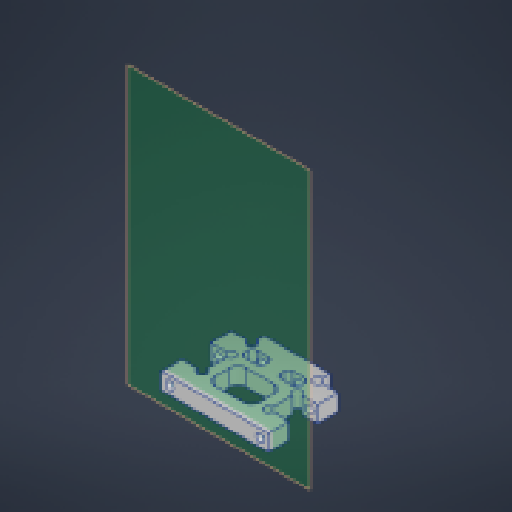
# Autodesk Inventor part: Roll_Fixation_Frameto64
Saved by Autodesk Inventor 2024 (Build 280153000, 153)
## iProperties
Created: 2024-01-23
Part Number: Roll_Fixation_Frameto64
Material: 알루미늄 6061
Document SubType Name: Modeling
Designer: ASUS
Density: 2.7 g/cm^3
Appearance: 알루미늄 - 평지
Author: ASUS
Autodesk Inventor part; units mm, degrees
ref_plane "작업 평면1" through (0, 37, 16) normal (0, 0, -1) x (-1, 0, 0)
sketch "스케치1" plane through (0, 37, 16) normal (0, 0, -1) x (-1, 0, 0)
  arc A0 (20.1, 4.5766) -> (19.5808, 6.2636) centre (17.1, 4.5766) ccw projected
  line L0 (19.5808, 6.2636) -> (15.5953, 12.1246) projected
  arc A1 (15.5953, 12.1246) -> (13.9414, 13) centre (13.9414, 11) ccw projected
  line L1 (13, 13) -> (13.9414, 13) projected
  arc A2 (14.5, 11.5) -> (13, 13) centre (13, 11.5) ccw projected
  line L2 (14.5, -41.5) -> (14.5, 11.5) projected
  arc A3 (13.5, -42.5) -> (14.5, -41.5) centre (13.5, -41.5) ccw projected
  line L3 (-13.5, -42.5) -> (13.5, -42.5) projected
  arc A4 (-14.5, -41.5) -> (-13.5, -42.5) centre (-13.5, -41.5) ccw projected
  line L4 (-14.5, 11.5) -> (-14.5, -41.5) projected
  arc A5 (-13, 13) -> (-14.5, 11.5) centre (-13, 11.5) ccw projected
  line L5 (-13.9414, 13) -> (-13, 13) projected
  arc A6 (-13.9414, 13) -> (-15.5953, 12.1246) centre (-13.9414, 11) ccw projected
  line L6 (-15.5953, 12.1246) -> (-19.5808, 6.2636) projected
  arc A7 (-19.5808, 6.2636) -> (-20.1, 4.5766) centre (-17.1, 4.5766) ccw projected
  line L7 (-20.1, 4.5766) -> (-20.1, -39.6766) projected
  arc A8 (-20.1, -39.6766) -> (-19.5808, -41.3636) centre (-17.1, -39.6766) ccw projected
  line L8 (-19.5808, -41.3636) -> (-15.8929, -46.7869) projected
  arc A9 (-15.8929, -46.7869) -> (-13.4121, -48.1) centre (-13.4121, -45.1) ccw projected
  line L9 (-13.4121, -48.1) -> (13.4121, -48.1) projected
  arc A10 (13.4121, -48.1) -> (15.8929, -46.7869) centre (13.4121, -45.1) ccw projected
  line L10 (15.8929, -46.7869) -> (19.5808, -41.3636) projected
  arc A11 (19.5808, -41.3636) -> (20.1, -39.6766) centre (17.1, -39.6766) ccw projected
  line L11 (20.1, -39.6766) -> (20.1, 4.5766) projected
  circle A12 centre (-17.3, 4) radius 1.35 projected
  circle A13 centre (-17.3, -18) radius 1.35 projected
  circle A14 centre (-11, -45.3) radius 1.35 projected
  circle A15 centre (17.3, 4) radius 1.35 projected
  circle A16 centre (17.3, -18) radius 1.35 projected
  circle A17 centre (11, -45.3) radius 1.35 projected
  circle A18 centre (-17.3, -40) radius 1.35 projected
  circle A19 centre (17.3, -40) radius 1.35 projected
  line L12 (-7.1991, -36.7384) -> (-5.2861, -28.9475) projected
  arc A20 (-2.675, -27.5395) -> (-5.2861, -28.9475) centre (-3.3438, -29.4244) ccw projected
  arc A21 (-2.675, -27.5395) -> (2.675, -27.5395) centre (0, -20) ccw projected
  arc A22 (5.2861, -28.9475) -> (2.675, -27.5395) centre (3.3438, -29.4244) ccw projected
  line L13 (5.2861, -28.9475) -> (7.1991, -36.7384) projected
  arc A23 (5.8409, -39.1281) -> (7.1991, -36.7384) centre (5.2568, -37.2153) ccw projected
  arc A24 (-5.8409, -39.1281) -> (5.8409, -39.1281) centre (0, -20) ccw projected
  arc A25 (-7.1991, -36.7384) -> (-5.8409, -39.1281) centre (-5.2568, -37.2153) ccw projected
  circle A26 centre (11, -45.3) radius 1.35 projected
  circle A27 centre (-11, -45.3) radius 1.35 projected
  arc A28 (-4, -43.3) -> (-8, -43.3) centre (-6, -43.3) ccw projected
  line L14 (-4, -43.3) -> (4, -43.3) projected
  arc A29 (8, -43.3) -> (4, -43.3) centre (6, -43.3) ccw projected
  line L15 (8, -43.3) -> (8, -47.3) projected
  arc A30 (4, -47.3) -> (8, -47.3) centre (6, -47.3) ccw projected
  line L16 (4, -47.3) -> (-4, -47.3) projected
  arc A31 (-8, -47.3) -> (-4, -47.3) centre (-6, -47.3) ccw projected
  line L17 (-8, -47.3) -> (-8, -43.3) projected
  line L18 (16.3659, -53.1031) -> (7.7692, -18.0923) projected
  arc A32 (7.7692, -18.0923) -> (-7.7692, -18.0923) centre (0, -20) ccw projected
  line L19 (-7.7692, -18.0923) -> (-16.3659, -53.1031) projected
  arc A33 (-16.3659, -53.1031) -> (-16.539, -54.5339) centre (-10.539, -54.5339) ccw projected
  line L20 (-16.539, -54.5339) -> (-16.539, -62.05) projected
  arc A34 (-16.539, -62.05) -> (-10.539, -68.05) centre (-10.539, -62.05) ccw projected
  line L21 (-10.539, -68.05) -> (10.539, -68.05) projected
  arc A35 (10.539, -68.05) -> (16.539, -62.05) centre (10.539, -62.05) ccw projected
  line L22 (16.539, -62.05) -> (16.539, -54.5339) projected
  arc A36 (16.539, -54.5339) -> (16.3659, -53.1031) centre (10.539, -54.5339) ccw projected
  circle A37 centre (10.539, -60) radius 1.35 projected
  circle A38 centre (-10.461, -60) radius 1.35 projected
  circle A39 centre (0, -20) radius 4 projected
  line L23 (-3.961, -62) -> (4.039, -62) projected
  arc A40 (-7.461, -62) -> (-3.961, -62) centre (-5.711, -62) ccw projected
  line L24 (-7.461, -58) -> (-7.461, -62) projected
  arc A41 (-3.961, -58) -> (-7.461, -58) centre (-5.711, -58) ccw projected
  line L25 (4.039, -58) -> (-3.961, -58) projected
  arc A42 (7.539, -58) -> (4.039, -58) centre (5.789, -58) ccw projected
  line L26 (7.539, -62) -> (7.539, -58) projected
  arc A43 (4.039, -62) -> (7.539, -62) centre (5.789, -62) ccw projected
  line L27 (13, -43.3) -> (9, -43.3)
  line L28 (9, -43.3) -> (9, -47.3)
  line L29 (9, -47.3) -> (13, -47.3)
  line L30 (13, -47.3) -> (13, -43.3)
  line L31 (13, -43.3) -> (9, -47.3) construction
  line L32 (9, -43.3) -> (13, -47.3) construction
  line L33 (-9, -43.3) -> (-13, -43.3)
  line L34 (-13, -43.3) -> (-13, -47.3)
  line L35 (-13, -47.3) -> (-9, -47.3)
  line L36 (-9, -47.3) -> (-9, -43.3)
  line L37 (-9, -43.3) -> (-13, -47.3) construction
  line L38 (-13, -43.3) -> (-9, -47.3) construction
  line L39 (13, -47.3) -> (-13, -47.3)
  line L40 (-13, -47.3) -> (-13, -43.3)
  line L41 (-13, -43.3) -> (13, -43.3)
  line L42 (13, -43.3) -> (13, -47.3)
  line L43 (4, -47.3) -> (-4, -47.3)
  line L44 (-4, -47.3) -> (-4, -43.3)
  line L45 (-4, -43.3) -> (4, -43.3)
  line L46 (4, -43.3) -> (4, -47.3)
  point P0 (0, -37)
  point P1 (4, -47.3)
  point P2 (4, -43.3)
  point P3 (-4, -43.3)
  dimension "d0" = 4
  dimension "d1" = 4
  dimension "d2" = 4
  dimension "d3" = 4
  constraints: 40 end point, 8 parallel, 4 horizontal, 4 midpoint, 4 perpendicular
  measures "d0" distance of L29.end L28.end
  measures "d1" distance of L28.end L27.end
  measures "d2" distance of L35.end L34.end
  measures "d3" distance of L34.end L33.end
ref_plane "작업 평면2" through (-16.539, -31.05, 0) normal (0, 0, 1) x (1, 0, 0)
extrude "돌출1" add sketch "스케치1" along normal up to surface (16 mm away) contours L39 L46 L41 L15 | L15 L41 L28 L39 | L16 L44 L14 L46 | L28 L27 L30 L29 | L39 L17 L41 L44 | L39 L36 L41 L17 | L35 L34 L33 L36
sketch "스케치2" plane through (13, -6.3, 0) normal (0, 0, -1) x (-1, 0, 0)
  line L0 (5.8009, 6.5616) -> (7.7139, 14.3525) projected
  arc A0 (10.325, 15.7605) -> (7.7139, 14.3525) centre (9.6562, 13.8756) ccw projected
  arc A1 (10.325, 15.7605) -> (15.675, 15.7605) centre (13, 23.3) ccw projected
  arc A2 (18.2861, 14.3525) -> (15.675, 15.7605) centre (16.3438, 13.8756) ccw projected
  line L1 (18.2861, 14.3525) -> (20.1991, 6.5616) projected
  arc A3 (18.8409, 4.1719) -> (20.1991, 6.5616) centre (18.2568, 6.0847) ccw projected
  arc A4 (7.1591, 4.1719) -> (18.8409, 4.1719) centre (13, 23.3) ccw projected
  arc A5 (5.8009, 6.5616) -> (7.1591, 4.1719) centre (7.7432, 6.0847) ccw projected
  circle A6 centre (24, -2) radius 1.35 projected
  circle A7 centre (2, -2) radius 1.35 projected
  arc A8 (9, 0) -> (5, 0) centre (7, 0) ccw projected
  line L2 (9, 0) -> (17, 0) projected
  arc A9 (21, 0) -> (17, 0) centre (19, 0) ccw projected
  line L3 (21, 0) -> (21, -4) projected
  arc A10 (17, -4) -> (21, -4) centre (19, -4) ccw projected
  line L4 (17, -4) -> (9, -4) projected
  arc A11 (5, -4) -> (9, -4) centre (7, -4) ccw projected
  line L5 (5, -4) -> (5, 0) projected
  line L6 (29.3659, -9.8031) -> (20.7692, 25.2077) projected
  arc A12 (20.7692, 25.2077) -> (5.2308, 25.2077) centre (13, 23.3) ccw projected
  line L7 (5.2308, 25.2077) -> (-3.3659, -9.8031) projected
  arc A13 (-3.3659, -9.8031) -> (-3.539, -11.2339) centre (2.461, -11.2339) ccw projected
  line L8 (-3.539, -11.2339) -> (-3.539, -18.75) projected
  arc A14 (-3.539, -18.75) -> (2.461, -24.75) centre (2.461, -18.75) ccw projected
  line L9 (2.461, -24.75) -> (23.539, -24.75) projected
  arc A15 (23.539, -24.75) -> (29.539, -18.75) centre (23.539, -18.75) ccw projected
  line L10 (29.539, -18.75) -> (29.539, -11.2339) projected
  arc A16 (29.539, -11.2339) -> (29.3659, -9.8031) centre (23.539, -11.2339) ccw projected
  circle A17 centre (23.539, -16.7) radius 1.35 projected
  circle A18 centre (2.539, -16.7) radius 1.35 projected
  circle A19 centre (13, 23.3) radius 4 projected
  line L11 (9.039, -18.7) -> (17.039, -18.7) projected
  arc A20 (5.539, -18.7) -> (9.039, -18.7) centre (7.289, -18.7) ccw projected
  line L12 (5.539, -14.7) -> (5.539, -18.7) projected
  arc A21 (9.039, -14.7) -> (5.539, -14.7) centre (7.289, -14.7) ccw projected
  line L13 (17.039, -14.7) -> (9.039, -14.7) projected
  arc A22 (20.539, -14.7) -> (17.039, -14.7) centre (18.789, -14.7) ccw projected
  line L14 (20.539, -18.7) -> (20.539, -14.7) projected
  arc A23 (17.039, -18.7) -> (20.539, -18.7) centre (18.789, -18.7) ccw projected
  line L15 (21, -4) -> (5, -4)
  line L16 (5, -4) -> (5, 0)
  line L17 (5, 0) -> (21, 0)
  line L18 (21, 0) -> (21, -4)
  point P0 (13, 6.3)
  point P1 (21, 0)
  point P2 (17, 0)
  point P3 (9, 0)
  point P4 (5, -4)
  point P5 (9, -4)
  point P6 (17, -4)
  constraints: 8 end point, 2 parallel, 1 horizontal, 1 perpendicular
ref_plane "작업 평면3" through (-16.539, -31.05, -2) normal (0, 0, -1) x (0, 1, 0)
extrude "돌출2" add sketch "스케치2" along normal up to surface (2 mm away) contours L2 L17 L3 L15 L4 L5
sketch "스케치3" plane through (-13, -10.3, 16) normal (0, -1, 0) x (1, 0, 0)
  line L0 (26, -16) -> (21, -16) projected
  line L1 (26, 0) -> (26, -16) projected
  line L2 (26, 0) -> (0, 0) projected
  line L3 (0, 0) -> (0, -16) projected
  line L4 (5, -16) -> (0, -16) projected
  line L5 (5, -16) -> (5, -18) projected
  line L6 (5, -18) -> (21, -18) projected
  line L7 (21, -16) -> (21, -18) projected
  circle A0 centre (5, -16) radius 1.1
  line L8 (21, -16) -> (21, -18) projected
  circle A1 centre (21, -16) radius 1.1
  point P0 (13, -16)
  dimension "d8" = 2.2
  dimension "d9" = 2.2
  constraints: 2 centre point, 2 coincident
  measures "d8" diameter of A0
  measures "d9" diameter of A1
extrude "돌출3" cut sketch "스케치3" against normal through all contours A1 L7 L0 | L0 L7 A1 | A0 L5 L4 | L4 L5 A0
sketch "스케치4" plane through (8, -6.3, -2) normal (0, 0, -1) x (-1, 0, 0)
  line L0 (16, 0) -> (16, -4) projected
  line L1 (0, 0) -> (16, 0) projected
  line L2 (0, -4) -> (0, 0) projected
  line L3 (16, -4) -> (0, -4) projected
  line L4 (16, -4) -> (16, 0) projected
  line L5 (16, -2) -> (0, -2)
  circle A0 centre (8, -2) radius 1
  circle A1 centre (8, -2) radius 2.5
  line L6 (17.1, -4) -> (14.9, -4) projected
  line L7 (1.1, -4) -> (-1.1, -4) projected
  line L8 (14.9, -4) -> (1.1, -4)
  line L9 (1.1, -4) -> (1.1, 0)
  line L10 (1.1, 0) -> (14.9, 0)
  line L11 (14.9, 0) -> (14.9, -4)
  line L12 (16, -4) -> (0, -4) projected
  circle A2 centre (-13.2666, 1.4722) radius 1
  circle A3 centre (-13.2666, 1.4722) radius 2.5
  line L13 (-13.2666, 1.4722) -> (-15.7666, 1.4722)
  line L14 (-13.2666, 1.4722) -> (-10.7666, 1.4722)
  circle A4 centre (14.9, -2) radius 0.5
  circle A5 centre (1.1, -2) radius 0.5
  circle A6 centre (12.4, -2) radius 1
  circle A7 centre (12.4, -2) radius 2.5
  line L15 (12.4, -2) -> (9.9, -2)
  line L16 (12.4, -2) -> (14.9, -2)
  circle A8 centre (3.6, -2) radius 1
  circle A9 centre (3.6, -2) radius 2.5
  line L17 (3.6, -2) -> (1.1, -2)
  line L18 (3.6, -2) -> (6.1, -2)
  point P0 (8, 6.3)
  dimension "d12" = 2
  dimension "d13" = 5
  dimension "d14" = 2
  dimension "d15" = 5
  dimension "d16" = 1
  dimension "d17" = 1
  dimension "d18" = 2
  dimension "d19" = 5
  dimension "d20" = 2
  dimension "d21" = 5
  constraints: 22 end point, 10 centre point, 6 horizontal, 6 point on circle, 5 midpoint, 4 coincident, 2 parallel, 1 collinear, 1 perpendicular
  measures "d12" diameter of A0
  measures "d13" diameter of A1
  measures "d14" diameter of A2
  measures "d15" diameter of A3
  measures "d16" diameter of A4
  measures "d17" diameter of A5
  measures "d18" diameter of A6
  measures "d19" diameter of A7
  measures "d20" diameter of A8
  measures "d21" diameter of A9
extrude "돌출4" cut sketch "스케치4" against normal blind 10 contours A6 L5 | L5 A6 | A8 L5 | L5 A8
sketch "스케치5" plane through (-13, -10.3, 0) normal (0, 0, -1) x (-1, 0, 0)
  circle A0 centre (-2, 2) radius 1.35 projected
  circle A1 centre (-24, 2) radius 1.35 projected
  line L0 (-20.1991, 10.5616) -> (-18.2861, 18.3525) projected
  arc A2 (-15.675, 19.7605) -> (-18.2861, 18.3525) centre (-16.3438, 17.8756) ccw projected
  arc A3 (-15.675, 19.7605) -> (-10.325, 19.7605) centre (-13, 27.3) ccw projected
  arc A4 (-7.7139, 18.3525) -> (-10.325, 19.7605) centre (-9.6562, 17.8756) ccw projected
  line L1 (-7.7139, 18.3525) -> (-5.8009, 10.5616) projected
  arc A5 (-7.1591, 8.1719) -> (-5.8009, 10.5616) centre (-7.7432, 10.0847) ccw projected
  arc A6 (-18.8409, 8.1719) -> (-7.1591, 8.1719) centre (-13, 27.3) ccw projected
  arc A7 (-20.1991, 10.5616) -> (-18.8409, 8.1719) centre (-18.2568, 10.0847) ccw projected
  circle A8 centre (-2, 2) radius 1.35 projected
  circle A9 centre (-24, 2) radius 1.35 projected
  arc A10 (-17, 4) -> (-21, 4) centre (-19, 4) ccw projected
  line L2 (-17, 4) -> (-9, 4) projected
  arc A11 (-5, 4) -> (-9, 4) centre (-7, 4) ccw projected
  line L3 (-5, 4) -> (-5, 0) projected
  arc A12 (-9, 0) -> (-5, 0) centre (-7, 0) ccw projected
  line L4 (-9, 0) -> (-17, 0) projected
  arc A13 (-21, 0) -> (-17, 0) centre (-19, 0) ccw projected
  line L5 (-21, 0) -> (-21, 4) projected
  line L6 (3.3659, -5.8031) -> (-5.2308, 29.2077) projected
  arc A14 (-5.2308, 29.2077) -> (-20.7692, 29.2077) centre (-13, 27.3) ccw projected
  line L7 (-20.7692, 29.2077) -> (-29.3659, -5.8031) projected
  arc A15 (-29.3659, -5.8031) -> (-29.539, -7.2339) centre (-23.539, -7.2339) ccw projected
  line L8 (-29.539, -7.2339) -> (-29.539, -14.75) projected
  arc A16 (-29.539, -14.75) -> (-23.539, -20.75) centre (-23.539, -14.75) ccw projected
  line L9 (-23.539, -20.75) -> (-2.461, -20.75) projected
  arc A17 (-2.461, -20.75) -> (3.539, -14.75) centre (-2.461, -14.75) ccw projected
  line L10 (3.539, -14.75) -> (3.539, -7.2339) projected
  arc A18 (3.539, -7.2339) -> (3.3659, -5.8031) centre (-2.461, -7.2339) ccw projected
  circle A19 centre (-2.461, -12.7) radius 1.35 projected
  circle A20 centre (-23.461, -12.7) radius 1.35 projected
  circle A21 centre (-13, 27.3) radius 4 projected
  line L11 (-16.961, -14.7) -> (-8.961, -14.7) projected
  arc A22 (-20.461, -14.7) -> (-16.961, -14.7) centre (-18.711, -14.7) ccw projected
  line L12 (-20.461, -10.7) -> (-20.461, -14.7) projected
  arc A23 (-16.961, -10.7) -> (-20.461, -10.7) centre (-18.711, -10.7) ccw projected
  line L13 (-8.961, -10.7) -> (-16.961, -10.7) projected
  arc A24 (-5.461, -10.7) -> (-8.961, -10.7) centre (-7.211, -10.7) ccw projected
  line L14 (-5.461, -14.7) -> (-5.461, -10.7) projected
  arc A25 (-8.961, -14.7) -> (-5.461, -14.7) centre (-7.211, -14.7) ccw projected
  circle A26 centre (-24, 2) radius 1
  circle A27 centre (-2, 2) radius 1
  point P0 (-13, 10.3)
  dimension "d24" = 2
  dimension "d25" = 2
  constraints: 2 centre point, 2 coincident
  measures "d24" diameter of A26
  measures "d25" diameter of A27
ref_plane "작업 평면4" through (-20.1, -11.1, 16) normal (0, 0, -1) x (0, 1, 0)
extrude "돌출5" add sketch "스케치5" against normal up to surface (16 mm away) contours A0 | A1
sketch "스케치6" plane through (-13, -10.3, 16) normal (0, -1, 0) x (1, 0, 0)
  arc A0 (22.1, -16) -> (21, -17.1) centre (21, -16) ccw projected
  line L0 (26, -16) -> (22.1, -16) projected
  line L1 (26, 0) -> (26, -16) projected
  line L2 (26, 0) -> (0, 0) projected
  line L3 (0, 0) -> (0, -16) projected
  line L4 (3.9, -16) -> (0, -16) projected
  arc A1 (5, -17.1) -> (3.9, -16) centre (5, -16) ccw projected
  line L5 (5, -17.1) -> (5, -18) projected
  line L6 (5, -18) -> (21, -18) projected
  line L7 (21, -17.1) -> (21, -18) projected
  line L8 (0, 0) -> (26, 0)
  line L9 (26, 0) -> (26, -16)
  line L10 (26, -16) -> (0, -16)
  line L11 (0, -16) -> (0, 0)
  line L12 (3.5, -12.5) -> (22.5, -12.5)
  line L13 (22.5, -12.5) -> (22.5, -3.5)
  line L14 (22.5, -3.5) -> (3.5, -3.5)
  line L15 (3.5, -3.5) -> (3.5, -12.5)
  point P0 (13, -16)
  dimension "d28" = 3.5
  constraints: 16 end point, 4 parallel, 2 perpendicular, 1 horizontal, 3 other
  measures "d28" distance between parallel lines of L10 L12
extrude "돌출6" cut sketch "스케치6" against normal through all contours L15 L14 L13 L12
sketch "스케치7" plane through (-13, -10.3, 16) normal (0, -1, 0) x (1, 0, 0)
  line L0 (3.5, -3.5) -> (22.5, -3.5) projected
  line L1 (22.5, -3.5) -> (22.5, -12.5) projected
  line L2 (22.5, -12.5) -> (3.5, -12.5) projected
  line L3 (3.5, -12.5) -> (3.5, -3.5) projected
  arc A0 (22.1, -16) -> (21, -17.1) centre (21, -16) ccw projected
  line L4 (26, -16) -> (22.1, -16) projected
  line L5 (26, 0) -> (26, -16) projected
  line L6 (26, 0) -> (0, 0) projected
  line L7 (0, 0) -> (0, -16) projected
  line L8 (3.9, -16) -> (0, -16) projected
  arc A1 (5, -17.1) -> (3.9, -16) centre (5, -16) ccw projected
  line L9 (5, -17.1) -> (5, -18) projected
  line L10 (5, -18) -> (21, -18) projected
  line L11 (21, -17.1) -> (21, -18) projected
  line L12 (3.5, -12.5) -> (13, -3.5)
  line L13 (22.5, -12.5) -> (13, -3.5)
  line L14 (4.1877, -13.226) -> (13, -4.8775)
  line L15 (13, -4.8775) -> (21.8123, -13.226)
  line L16 (2.8123, -11.774) -> (13, -2.1225)
  line L17 (13, -2.1225) -> (23.1877, -11.774)
  point P0 (13, -16)
  point P1 (11.546, -3.5)
  point P2 (3.5, -11.1225)
  point P3 (4.954, -12.5)
  point P4 (21.046, -12.5)
  point P5 (22.5, -11.1225)
  point P6 (14.454, -3.5)
  dimension "d31" = 1
  dimension "d32" = 1
  constraints: 12 end point, 1 midpoint, 2 other
  measures "d31" distance between parallel lines of L12 L14
  measures "d32" distance between parallel lines of L12 L16
extrude "돌출7" add sketch "스케치7" against normal up to surface (4 mm away) contours L0 L12 L3 L16 | L13 L2 L15 L14 L12 | L0 L17 L1 L13
fillet "모깎기1" radius 1 9 edges at (-9.5, -8.3, 12.5) (-9.5, -8.3, 4.8775) (-1.454, -8.3, 12.5) (0, -8.3, 11.1225) (1.454, -8.3, 12.5) (9.5, -8.3, 12.5) (9.5, -8.3, 4.8775) (8.046, -8.3, 3.5) (-8.046, -8.3, 3.5)
sketch "스케치8" plane through (0, 37, 16) normal (0, 0, 1) x (1, 0, 0)
  circle A0 centre (11, -45.3) radius 1 projected
  circle A1 centre (-11, -45.3) radius 1 projected
  line L0 (-13, -43.3) -> (13, -43.3) projected
  line L1 (-13, -47.3) -> (-13, -43.3) projected
  line L2 (13, -47.3) -> (-13, -47.3) projected
  line L3 (13, -43.3) -> (13, -47.3) projected
  point P0 (0, -37)
extrude "돌출8" add sketch "스케치8" along normal blind 1
sketch "스케치9" plane through (8, -6.3, -2) normal (0, 0, -1) x (-1, 0, 0)
  circle A0 centre (3.6, -2) radius 1 projected
  circle A1 centre (12.4, -2) radius 1 projected
  line L0 (16, 0) -> (16, -4) projected
  line L1 (0, 0) -> (16, 0) projected
  line L2 (0, -4) -> (0, 0) projected
  line L3 (16, -4) -> (0, -4) projected
  point P0 (8, 6.3)
ref_plane "작업 평면5" through (-21.6156, -28.6331, -3) normal (0, 0, -1) x (0, 1, 0)
extrude "돌출9" add sketch "스케치9" along normal up to surface (1 mm away)
sketch "스케치10" plane through (9.1, -10.3, 0) normal (0, -1, 0) x (1, 0, 0)
  line L0 (-5.1364, 12.5) -> (-0.6, 12.5) projected
  arc A0 (0.4, 11.5) -> (-0.6, 12.5) centre (-0.6, 11.5) ccw projected
  line L1 (0.4, 11.5) -> (0.4, 7.2024) projected
  arc A1 (-1.2877, 6.4764) -> (0.4, 7.2024) centre (-0.6, 7.2024) ccw projected
  line L2 (-1.2877, 6.4764) -> (-5.8241, 10.774) projected
  arc A2 (-5.1364, 12.5) -> (-5.8241, 10.774) centre (-5.1364, 11.5) ccw projected
  line L3 (-12.3759, 10.774) -> (-16.9123, 6.4764) projected
  arc A3 (-18.6, 7.2024) -> (-16.9123, 6.4764) centre (-17.6, 7.2024) ccw projected
  line L4 (-18.6, 7.2024) -> (-18.6, 11.5) projected
  arc A4 (-17.6, 12.5) -> (-18.6, 11.5) centre (-17.6, 11.5) ccw projected
  line L5 (-17.6, 12.5) -> (-13.0636, 12.5) projected
  arc A5 (-12.3759, 10.774) -> (-13.0636, 12.5) centre (-13.0636, 11.5) ccw projected
  line L6 (-15.3241, 5.226) -> (-9.7877, 10.471) projected
  arc A6 (-8.4123, 10.471) -> (-9.7877, 10.471) centre (-9.1, 9.745) ccw projected
  line L7 (-8.4123, 10.471) -> (-2.8759, 5.226) projected
  arc A7 (-3.5636, 3.5) -> (-2.8759, 5.226) centre (-3.5636, 4.5) ccw projected
  line L8 (-3.5636, 3.5) -> (-14.6364, 3.5) projected
  arc A8 (-15.3241, 5.226) -> (-14.6364, 3.5) centre (-14.6364, 4.5) ccw projected
  arc A9 (0, 0) -> (-1.1, -1.1) centre (-1.1, 0) ccw projected
  line L9 (3.9, 0) -> (0, 0) projected
  line L10 (3.9, 17) -> (3.9, 0) projected
  line L11 (-22.1, 17) -> (3.9, 17) projected
  line L12 (-22.1, 17) -> (-22.1, 0) projected
  line L13 (-18.2, 0) -> (-22.1, 0) projected
  arc A10 (-17.1, -1.1) -> (-18.2, 0) centre (-17.1, 0) ccw projected
  line L14 (-17.1, -1.1) -> (-17.1, -3) projected
  line L15 (-17.1, -3) -> (-1.1, -3) projected
  line L16 (-1.1, -1.1) -> (-1.1, -3) projected
  point P0 (-9.1, 0)
extrude "돌출10" add sketch "스케치10" against normal up to surface (4 mm away) contours L0 A0 L1 A1 L2 A2 | L3 A3 L4 A4 L5 A5 | L6 A6 L7 A7 L8 A8
sketch "스케치11" plane through (9.1, -10.3, 0) normal (0, -1, 0) x (1, 0, 0)
  line L0 (-19.1, 0) -> (-21.1, 0) projected
  line L1 (2.9, 0) -> (0.9, 0) projected
  arc A0 (0, 0) -> (-1.1, -1.1) centre (-1.1, 0) ccw projected
  line L2 (3.9, 0) -> (0, 0) projected
  line L3 (3.9, 17) -> (3.9, 0) projected
  line L4 (-22.1, 17) -> (3.9, 17) projected
  line L5 (-22.1, 17) -> (-22.1, 0) projected
  line L6 (-18.2, 0) -> (-22.1, 0) projected
  arc A1 (-17.1, -1.1) -> (-18.2, 0) centre (-17.1, 0) ccw projected
  line L7 (-17.1, -1.1) -> (-17.1, -3) projected
  line L8 (-17.1, -3) -> (-1.1, -3) projected
  line L9 (-1.1, -1.1) -> (-1.1, -3) projected
  line L10 (-22.1, 17) -> (-22.1, 0) projected
  line L11 (-22.1, 17) -> (-22.1, 0)
  line L12 (-22.1, 0) -> (-20.1, 0)
  line L13 (-20.1, 0) -> (-20.1, 17)
  line L14 (-20.1, 17) -> (-22.1, 17)
  line L15 (3.9, 17) -> (3.9, 0)
  line L16 (3.9, 0) -> (1.9, 0)
  line L17 (1.9, 0) -> (1.9, 17)
  line L18 (1.9, 17) -> (3.9, 17)
  line L19 (-22.1, 0) -> (-20.1, 0)
  line L20 (-20.1, 0) -> (-20.1, 5)
  line L21 (-20.1, 5) -> (-22.1, 5)
  line L22 (-22.1, 5) -> (-22.1, 0)
  line L23 (-22.1, 17) -> (3.9, 17) projected
  line L24 (-20.1, 17) -> (-22.1, 17)
  line L25 (-22.1, 17) -> (-22.1, 12)
  line L26 (-22.1, 12) -> (-20.1, 12)
  line L27 (-20.1, 12) -> (-20.1, 17)
  line L28 (1.9, 17) -> (3.9, 17)
  line L29 (3.9, 17) -> (3.9, 12)
  line L30 (3.9, 12) -> (1.9, 12)
  line L31 (1.9, 12) -> (1.9, 17)
  line L32 (1.9, 0) -> (3.9, 0)
  line L33 (3.9, 0) -> (3.9, 5)
  line L34 (3.9, 5) -> (1.9, 5)
  line L35 (1.9, 5) -> (1.9, 0)
  line L36 (-18.1, 10.5) -> (-22.1, 10.5)
  line L37 (-22.1, 10.5) -> (-22.1, 13.5)
  line L38 (-22.1, 13.5) -> (-18.1, 13.5)
  line L39 (-18.1, 13.5) -> (-18.1, 10.5)
  line L40 (-18.1, 10.5) -> (-22.1, 13.5) construction
  line L41 (-22.1, 10.5) -> (-18.1, 13.5) construction
  line L42 (-22.1, 5) -> (-20.1, 5)
  line L43 (-18.1, 3.5) -> (-22.1, 3.5)
  line L44 (-22.1, 3.5) -> (-22.1, 6.5)
  line L45 (-22.1, 6.5) -> (-18.1, 6.5)
  line L46 (-18.1, 6.5) -> (-18.1, 3.5)
  line L47 (-18.1, 3.5) -> (-22.1, 6.5) construction
  line L48 (-22.1, 3.5) -> (-18.1, 6.5) construction
  line L49 (-0.1, 5) -> (1.9, 5)
  line L50 (3.9, 3.5) -> (-0.1, 3.5)
  line L51 (-0.1, 3.5) -> (-0.1, 6.5)
  line L52 (-0.1, 6.5) -> (3.9, 6.5)
  line L53 (3.9, 6.5) -> (3.9, 3.5)
  line L54 (3.9, 3.5) -> (-0.1, 6.5) construction
  line L55 (-0.1, 3.5) -> (3.9, 6.5) construction
  line L56 (-0.1, 12) -> (1.9, 12)
  line L57 (3.9, 10.5) -> (-0.1, 10.5)
  line L58 (-0.1, 10.5) -> (-0.1, 13.5)
  line L59 (-0.1, 13.5) -> (3.9, 13.5)
  line L60 (3.9, 13.5) -> (3.9, 10.5)
  line L61 (3.9, 10.5) -> (-0.1, 13.5) construction
  line L62 (-0.1, 10.5) -> (3.9, 13.5) construction
  line L63 (-22.1, 13.5) -> (-22.1, 10.5)
  line L64 (-22.1, 10.5) -> (-17.1, 10.5)
  line L65 (-17.1, 10.5) -> (-17.1, 13.5)
  line L66 (-17.1, 13.5) -> (-22.1, 13.5)
  line L67 (-22.1, 6.5) -> (-22.1, 3.5)
  line L68 (-22.1, 3.5) -> (3.9, 3.5)
  line L69 (3.9, 3.5) -> (3.9, 6.5)
  line L70 (3.9, 6.5) -> (-22.1, 6.5)
  line L71 (3.9, 3.5) -> (3.9, 6.5)
  line L72 (3.9, 6.5) -> (-1.1, 6.5)
  line L73 (-1.1, 6.5) -> (-1.1, 3.5)
  line L74 (-1.1, 3.5) -> (3.9, 3.5)
  line L75 (3.9, 13.5) -> (3.9, 10.5)
  line L76 (3.9, 10.5) -> (-1.1, 10.5)
  line L77 (-1.1, 10.5) -> (-1.1, 13.5)
  line L78 (-1.1, 13.5) -> (3.9, 13.5)
  line L79 (-17.1, 13.5) -> (-1.1, 13.5)
  line L80 (-1.1, 13.5) -> (-1.1, 3.5)
  line L81 (-1.1, 3.5) -> (-17.1, 3.5)
  line L82 (-17.1, 3.5) -> (-17.1, 13.5)
  line L83 (-22.1, 12) -> (3.9, 12)
  line L84 (3.9, 12) -> (3.9, 5)
  line L85 (3.9, 5) -> (-22.1, 5)
  line L86 (-22.1, 5) -> (-22.1, 12)
  point P0 (-9.1, 0)
  point P1 (-1.1, 12)
  point P2 (-1.1, 10.5)
  point P3 (-1.1, 6.5)
  point P4 (-1.1, 5)
  point P5 (1.9, 5)
  point P6 (3.9, 5)
  point P7 (3.9, 12)
  point P8 (1.9, 12)
  point P9 (-17.1, 5)
  point P10 (-17.1, 12)
  point P11 (-22.1, 12)
  dimension "d42" = 2
  dimension "d43" = 2
  dimension "d44" = 5
  dimension "d45" = 5
  dimension "d46" = 5
  dimension "d47" = 5
  dimension "d48" = 3
  dimension "d49" = 3
  dimension "d50" = 3
  dimension "d51" = 3
  dimension "d52" = 5
  dimension "d53" = 5
  dimension "d54" = 5
  constraints: 150 end point, 32 parallel, 20 perpendicular, 8 midpoint, 6 collinear, 6 horizontal, 1 point on line
  measures "d42" distance of L12.end L5.end
  measures "d43" distance of L2.start L16.end
  measures "d44" distance of L20.end L12.end
  measures "d45" distance of L25.end L4.start
  measures "d46" distance of L3.start L29.end
  measures "d47" distance of L33.end L2.start
  measures "d48" distance of L36.end L37.end
  measures "d49" distance of L43.end L45.start
  measures "d50" distance of L50.end L52.start
  measures "d51" distance of L57.end L59.start
  measures "d52" distance of L64.end L36.end
  measures "d53" distance of L72.end L69.end
  measures "d54" distance of L57.start L76.end
extrude "돌출11" cut sketch "스케치11" against normal through all contours L21 L5 L45 L13 | L13 L45 L46 L85 | L45 L5 L36 L13 | L13 L36 L64 L82 L70 L45 | L46 L70 L82 L85 | L36 L5 L26 L13 | L13 L83 L39 L36 | L39 L83 L65 L64 | L73 L70 L51 L85 | L80 L76 L57 L17 L52 L70 | L51 L52 L17 L49 | L77 L83 L58 L76 | L17 L52 L3 L34 | L17 L57 L3 L52 | L58 L56 L17 L57 | L17 L30 L3 L57
sketch "스케치12" plane through (-13, -10.3, 0) normal (0, -1, 0) x (1, 0, 0)
  line L0 (21, 12) -> (26, 12) projected
  line L1 (26, 17) -> (26, 12) projected
  line L2 (0, 17) -> (26, 17) projected
  line L3 (0, 17) -> (0, 12) projected
  line L4 (0, 12) -> (5, 12) projected
  line L5 (5, 12) -> (5, 5) projected
  line L6 (5, 5) -> (0, 5) projected
  line L7 (0, 5) -> (0, 0) projected
  line L8 (3.9, 0) -> (0, 0) projected
  arc A0 (5, -1.1) -> (3.9, 0) centre (5, 0) ccw projected
  line L9 (5, -1.1) -> (5, -3) projected
  line L10 (5, -3) -> (21, -3) projected
  line L11 (21, -1.1) -> (21, -3) projected
  arc A1 (22.1, 0) -> (21, -1.1) centre (21, 0) ccw projected
  line L12 (26, 0) -> (22.1, 0) projected
  line L13 (26, 5) -> (26, 0) projected
  line L14 (26, 5) -> (21, 5) projected
  line L15 (21, 5) -> (21, 12) projected
  circle A2 centre (5, 12) radius 1.1
  circle A3 centre (5, 5) radius 1.1
  circle A4 centre (21, 5) radius 1.1
  circle A5 centre (21, 12) radius 1.1
  point P0 (13, 0)
  dimension "d57" = 2.2
  dimension "d58" = 2.2
  dimension "d59" = 2.2
  dimension "d60" = 2.2
  constraints: 4 centre point, 4 coincident
  measures "d57" diameter of A2
  measures "d58" diameter of A3
  measures "d59" diameter of A4
  measures "d60" diameter of A5
extrude "돌출12" cut sketch "스케치12" against normal through all contours L15 A5 L0 | L0 A5 L15 | A4 L14 L15 | L15 L14 A4 | A2 L5 L4 | L4 L5 A2 | A3 L6 L5 | L5 L6 A3
sketch "스케치13" plane through (-13, -10.3, 0) normal (0, -1, 0) x (1, 0, 0)
  line L0 (7.6, -3) -> (9.6, -3) projected
  line L1 (16.4, -3) -> (18.4, -3) projected
  line L2 (0, 17) -> (26, 17) projected
  line L3 (8.6, -3) -> (8.6, 17)
  line L4 (8.6, 17) -> (17.4, 17)
  line L5 (17.4, 17) -> (17.4, -3)
  line L6 (17.4, -3) -> (8.6, -3)
  arc A0 (22.1, 12) -> (21, 10.9) centre (21, 12) ccw projected
  line L7 (22.1, 12) -> (26, 12) projected
  line L8 (26, 17) -> (26, 12) projected
  line L9 (0, 17) -> (26, 17) projected
  line L10 (0, 17) -> (0, 12) projected
  line L11 (0, 12) -> (3.9, 12) projected
  arc A1 (5, 10.9) -> (3.9, 12) centre (5, 12) ccw projected
  line L12 (5, 10.9) -> (5, 6.1) projected
  arc A2 (3.9, 5) -> (5, 6.1) centre (5, 5) ccw projected
  line L13 (3.9, 5) -> (0, 5) projected
  line L14 (0, 5) -> (0, 0) projected
  line L15 (3.9, 0) -> (0, 0) projected
  arc A3 (5, -1.1) -> (3.9, 0) centre (5, 0) ccw projected
  line L16 (5, -1.1) -> (5, -3) projected
  line L17 (5, -3) -> (21, -3) projected
  line L18 (21, -1.1) -> (21, -3) projected
  arc A4 (22.1, 0) -> (21, -1.1) centre (21, 0) ccw projected
  line L19 (26, 0) -> (22.1, 0) projected
  line L20 (26, 5) -> (26, 0) projected
  line L21 (26, 5) -> (22.1, 5) projected
  arc A5 (21, 6.1) -> (22.1, 5) centre (21, 5) ccw projected
  line L22 (21, 6.1) -> (21, 10.9) projected
  line L23 (5, 10.9) -> (5, 6.1) projected
  line L24 (5, 8.5) -> (21, 8.5)
  line L25 (0, 2.5) -> (26, 2.5)
  line L26 (6.1, 1) -> (11.1, 1)
  line L27 (11.1, 1) -> (11.1, 4)
  line L28 (11.1, 4) -> (6.1, 4)
  line L29 (6.1, 4) -> (6.1, 1)
  line L30 (6.1, 1) -> (11.1, 4) construction
  line L31 (11.1, 1) -> (6.1, 4) construction
  line L32 (14.9, 1) -> (19.9, 1)
  line L33 (19.9, 1) -> (19.9, 4)
  line L34 (19.9, 4) -> (14.9, 4)
  line L35 (14.9, 4) -> (14.9, 1)
  line L36 (14.9, 1) -> (19.9, 4) construction
  line L37 (19.9, 1) -> (14.9, 4) construction
  point P0 (13, 0)
  point P1 (8.6, 2.5)
  point P2 (17.4, 2.5)
  dimension "d63" = 5
  dimension "d64" = 3
  dimension "d65" = 5
  dimension "d66" = 3
  constraints: 36 end point, 9 midpoint, 6 parallel, 5 point on line, 3 perpendicular, 2 horizontal, 1 vertical
  measures "d63" distance of L28.end L27.end
  measures "d64" distance of L27.end L26.end
  measures "d65" distance of L34.end L33.end
  measures "d66" distance of L33.end L32.end
extrude "돌출13" cut sketch "스케치13" against normal through all contours L26 L29 L25 L3 | L3 L25 L27 L26 | L25 L29 L28 L3 | L3 L28 L27 L25 | L32 L35 L25 L5 | L5 L25 L33 L32 | L35 L34 L5 L25 | L5 L34 L33 L25
fillet "모깎기2" radius 1 8 edges at (-6.9, -8.3, 4) (-6.9, -8.3, 1) (-1.9, -8.3, 1) (-1.9, -8.3, 4) (1.9, -8.3, 4) (1.9, -8.3, 1) (6.9, -8.3, 1) (6.9, -8.3, 4)
sketch "스케치14" plane through (-13, -10.3, 0) normal (0, -1, 0) x (1, 0, 0)
  line L0 (18.9, 1) -> (15.9, 1) projected
  arc A0 (14.9, 2) -> (15.9, 1) centre (15.9, 2) ccw projected
  line L1 (14.9, 2) -> (14.9, 3) projected
  arc A1 (15.9, 4) -> (14.9, 3) centre (15.9, 3) ccw projected
  line L2 (15.9, 4) -> (18.9, 4) projected
  arc A2 (19.9, 3) -> (18.9, 4) centre (18.9, 3) ccw projected
  line L3 (19.9, 3) -> (19.9, 2) projected
  arc A3 (18.9, 1) -> (19.9, 2) centre (18.9, 2) ccw projected
  line L4 (11.1, 3) -> (11.1, 2) projected
  arc A4 (10.1, 1) -> (11.1, 2) centre (10.1, 2) ccw projected
  line L5 (10.1, 1) -> (7.1, 1) projected
  arc A5 (6.1, 2) -> (7.1, 1) centre (7.1, 2) ccw projected
  line L6 (6.1, 2) -> (6.1, 3) projected
  arc A6 (7.1, 4) -> (6.1, 3) centre (7.1, 3) ccw projected
  line L7 (7.1, 4) -> (10.1, 4) projected
  arc A7 (11.1, 3) -> (10.1, 4) centre (10.1, 3) ccw projected
  arc A8 (22.1, 12) -> (21, 10.9) centre (21, 12) ccw projected
  line L8 (22.1, 12) -> (26, 12) projected
  line L9 (26, 17) -> (26, 12) projected
  line L10 (0, 17) -> (26, 17) projected
  line L11 (0, 17) -> (0, 12) projected
  line L12 (0, 12) -> (3.9, 12) projected
  arc A9 (5, 10.9) -> (3.9, 12) centre (5, 12) ccw projected
  line L13 (5, 10.9) -> (5, 6.1) projected
  arc A10 (3.9, 5) -> (5, 6.1) centre (5, 5) ccw projected
  line L14 (3.9, 5) -> (0, 5) projected
  line L15 (0, 5) -> (0, 0) projected
  line L16 (3.9, 0) -> (0, 0) projected
  arc A11 (5, -1.1) -> (3.9, 0) centre (5, 0) ccw projected
  line L17 (5, -1.1) -> (5, -3) projected
  line L18 (5, -3) -> (21, -3) projected
  line L19 (21, -1.1) -> (21, -3) projected
  arc A12 (22.1, 0) -> (21, -1.1) centre (21, 0) ccw projected
  line L20 (26, 0) -> (22.1, 0) projected
  line L21 (26, 5) -> (26, 0) projected
  line L22 (26, 5) -> (22.1, 5) projected
  arc A13 (21, 6.1) -> (22.1, 5) centre (21, 5) ccw projected
  line L23 (21, 6.1) -> (21, 10.9) projected
  line L24 (19.9, 3) -> (6.1, 3)
  line L25 (6.1, 3) -> (6.1, 15)
  line L26 (6.1, 15) -> (19.9, 15)
  line L27 (19.9, 15) -> (19.9, 3)
  line L28 (18.4, 4.5) -> (7.6, 4.5)
  line L29 (7.6, 4.5) -> (7.6, 13.5)
  line L30 (7.6, 13.5) -> (18.4, 13.5)
  line L31 (18.4, 13.5) -> (18.4, 4.5)
  line L32 (18.4, 4.5) -> (7.6, 4.5)
  line L33 (7.6, 4.5) -> (7.6, 6)
  line L34 (7.6, 6) -> (18.4, 6)
  line L35 (18.4, 6) -> (18.4, 4.5)
  point P0 (13, 0)
  point P1 (7.6, 6)
  dimension "d70" = 12
  dimension "d71" = 1.5
  dimension "d72" = 1.5
  constraints: 24 end point, 7 equal length, 3 perpendicular, 1 horizontal, 3 other
  measures "d70" distance of L6.end L25.end
  measures "d71" distance between parallel lines of L27 L31
  measures "d72" distance of L28.end L33.end
extrude "돌출14" cut sketch "스케치14" against normal through all contours L34 L29 L30 L31
fillet "모깎기3" radius 2 4 edges at (5.4, -8.3, 13.5) (5.4, -8.3, 6) (-5.4, -8.3, 6) (-5.4, -8.3, 13.5)
